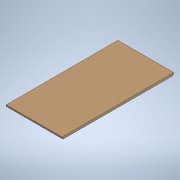
# Autodesk Inventor part: desk
Saved by Autodesk Inventor 2022 (Build 260153000, 153)
## iProperties
Created: 2022-02-21
Part Number: desk
Material: MDF Medium Density Fiberboard
Document SubType Name: Modeling
Designer: MarkP
Density: 0.8 g/cm^3
Appearance: Cardboard - Corrugated
Author: MarkP
Autodesk Inventor part; units mm, degrees
ref_plane "YZ Plane" through (0, 0, 0) normal (1, 0, 0) x (0, 1, 0)
ref_plane "XZ Plane" through (0, 0, 0) normal (0, 1, 0) x (-1, 0, 0)
ref_plane "XY Plane" through (0, 0, 0) normal (0, 0, 1) x (1, 0, 0)
sketch "Sketch1" plane through (0, 0, 0) normal (0, 1, 0) x (-1, 0, 0)
  line L0 (0, 0) -> (750, 0)
  line L1 (750, 0) -> (750, -1500)
  line L2 (750, -1500) -> (0, -1500)
  line L3 (0, -1500) -> (0, 0)
  dimension "d0" = 750
  dimension "d1" = 1500
  constraints: 8 end point, 2 parallel, 1 horizontal, 1 perpendicular
  measures "d0" distance of L1.end L2.end
  measures "d1" distance of L0.end L1.end
extrude "Extrusion1" add sketch "Sketch1" along normal blind 32
sketch "Sketch3" plane through (0, 0, 0) normal (0, -1, 0) x (1, 0, 0)
  line L0 (-750, 0) -> (0, 0) projected
  line L1 (-750, -1500) -> (-750, 0) projected
  line L2 (0, 0) -> (-750, 0)
  line L3 (-750, 0) -> (-750, -12)
  line L4 (-750, -12) -> (0, -12)
  line L5 (0, -12) -> (0, 0)
  line L6 (0, -1500) -> (-750, -1500) projected
  line L7 (0, 0) -> (0, -1500) projected
  line L8 (-750, -1500) -> (0, -1500)
  line L9 (0, -1500) -> (0, -1488)
  line L10 (0, -1488) -> (-750, -1488)
  line L11 (-750, -1488) -> (-750, -1500)
  dimension "d4" = 12
  dimension "d5" = 12
  constraints: 16 end point, 4 parallel, 2 horizontal, 2 perpendicular, 2 point on line
  measures "d4" distance of L3.end L2.end
  measures "d5" distance of L9.end L8.end
extrude "Extrusion2" cut sketch "Sketch3" against normal blind 12 contours L0 L5 L4 L1 | L10 L7 L6 L1
body "Solid1"
